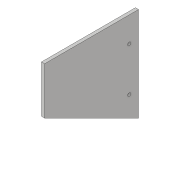
# Autodesk Inventor part: rudder
Saved by Autodesk Inventor 2020 (Build 240168000, 168)
## iProperties
Created: 2019-12-24
Part Number: rudder
Material: Generic
Document SubType Name: Sheet Metal
Designer: alifhabib
Density: 1 g/cm^3
Sheet Metal Rule: Default_mm
Appearance: Default
Author: alifhabib
Autodesk Inventor part; units mm, degrees
ref_plane "YZ Plane" through (0, 0, 0) normal (1, 0, 0) x (0, 1, 0)
ref_plane "XZ Plane" through (0, 0, 0) normal (0, 1, 0) x (-1, 0, 0)
ref_plane "XY Plane" through (0, 0, 0) normal (0, 0, 1) x (1, 0, 0)
sketch "Sketch1" plane through (0, 0, 0) normal (1, 0, 0) x (0, 1, 0)
  line L0 (0, 0) -> (661.0386, 0)
  line L1 (661.0386, 0) -> (661.0386, 150)
  line L2 (661.0386, 0) -> (511.0386, 0)
  line L3 (661.0386, 150) -> (586.0386, 150)
  line L4 (586.0386, 150) -> (511.0386, 0)
  point P0 (0, 0)
  dimension "d0" = 150
  dimension "d1" = 150
  dimension "d2" = 75
  measures "d0" distance of L0.end L1.end
  measures "d1" distance of L0.end L2.end
  measures "d2" distance of L1.end L3.end
extrude "Plate1" add sketch "Sketch1" along normal blind 5
sketch "Sketch2" plane through (5, 0, 0) normal (1, 0, 0) x (0, 0, -1)
  line L0 (-150, 661.0386) -> (0, 661.0386) projected
  line L1 (0, 661.0386) -> (0, 511.0386) projected
  circle A0 centre (-15, 621.0386) radius 2.5
  line L2 (0, 511.0386) -> (0, 661.0386) projected
  line L3 (0, 586.0386) -> (-15, 586.0386)
  circle A1 centre (-15, 551.0386) radius 2.5
  point P0 (0, 0)
  dimension "d4" = 40
  dimension "d5" = 15
  dimension "d6" = 5
  constraints: 2 centre point, 2 coincident, 2 end point, 2 symmetric about line, 1 horizontal, 1 midpoint, 1 other
  measures "d4" distance from line of L0 point (-15, 621.039)
  measures "d5" distance from line of L1 point (-15, 621.039)
  measures "d6" diameter of A0
extrude "Extrusion1" cut sketch "Sketch2" along normal mid plane 10
equation "\"d3\" = Thickness"
equation "\"BendRadius\" = Thickness"
equation "\"BendReliefWidth\" = Thickness"
equation "\"BendReliefDepth\" = 0.5 * Thickness"
equation "\"TransitionRadius\" = BendRadius"
equation "\"JacobiRadiusSize\" = BendRadius"
equation "\"GapSize\" = Thickness"
equation "\"Thickness\" = 5"
body "Solid1"
